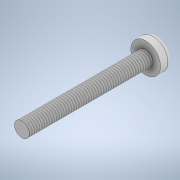
# Autodesk Inventor part: 16x2.5 Bolt
Saved by Autodesk Inventor 2022 (Build 260153000, 153)
## iProperties
Created: 2022-03-31
Part Number: 16x2.5 Bolt
Material: Generic
Document SubType Name: Modeling
Designer: Seppe
Density: 1 g/cm^3
Appearance: Default
Author: Seppe
Autodesk Inventor part; units mm, degrees
ref_plane "YZ Plane" through (0, 0, 0) normal (1, 0, 0) x (0, 1, 0)
ref_plane "XZ Plane" through (0, 0, 0) normal (0, 1, 0) x (-1, 0, 0)
ref_plane "XY Plane" through (0, 0, 0) normal (0, 0, 1) x (1, 0, 0)
sketch "Sketch1" plane through (0, 0, 0) normal (0, 0, 1) x (1, 0, 0)
  circle A0 centre (0, 0) radius 1.5
  circle A1 centre (0, 0) radius 3
  dimension "d0" = 3
  dimension "d1" = 6
  constraints: 2 centre point, 2 coincident
  measures "d0" diameter of A0
  measures "d1" diameter of A1
extrude "Extrusion1" add sketch "Sketch1" along normal blind 25 contours A0
sketch "Sketch2" plane through (0, 0, 0) normal (0, 0, -1) x (-1, 0, 0)
  point P0 (0, 0)
extrude "Extrusion2" add sketch "Sketch1" against normal blind 2.5 contours A0 | A1
thread "Thread1" size "M3x0.5" class "6g" standard "ISO Metric profile" full length
sketch "Sketch3" plane through (0, 0, -2.5) normal (0, 0, -1) x (-1, 0, 0)
  point P0 (0, 0)
sketch "Sketch4" plane through (0, 0, -2.5) normal (0, 0, -1) x (-1, 0, 0)
  line L0 (-0.5, -2) -> (0.5, -2)
  line L1 (0.5, -2) -> (0.5, 2)
  line L2 (0.5, 2) -> (-0.5, 2)
  line L3 (-0.5, 2) -> (-0.5, -2)
  circle A0 centre (0, 0) radius 1.5 projected
  line L4 (-0.5, -2) -> (0.5, 2) construction
  line L5 (0.5, -2) -> (-0.5, 2) construction
  line L6 (-2, -0.5) -> (2, -0.5)
  line L7 (2, -0.5) -> (2, 0.5)
  line L8 (2, 0.5) -> (-2, 0.5)
  line L9 (-2, 0.5) -> (-2, -0.5)
  circle A1 centre (0, 0) radius 3 projected
  line L10 (-2, -0.5) -> (2, 0.5) construction
  line L11 (2, -0.5) -> (-2, 0.5) construction
  point P0 (-0.5, 0.5)
  point P1 (-0.5, -0.5)
  point P2 (0.5, -0.5)
  point P3 (0.5, 0.5)
  dimension "d8" = 1
  dimension "d9" = 4
  dimension "d10" = 4
  dimension "d11" = 1
  constraints: 24 end point, 4 midpoint, 4 parallel, 2 horizontal, 2 perpendicular
  measures "d8" distance of L2.end L1.end
  measures "d9" distance of L1.end L0.end
  measures "d10" distance of L8.end L7.end
  measures "d11" distance of L7.end L6.end
extrude "Extrusion3" cut sketch "Sketch4" against normal blind 1 contours L3 A0 L1 L0 | L3 L6 L1 A0 | L6 A0 L8 L3 | L3 L8 L1 L6 | L6 L9 L8 A0 | L1 L8 A0 L6 | A0 L8 L7 L6 | L3 A0 L1 L8 | L3 L2 L1 A0
fillet "Fillet1" radius 1 1 edges at (-3, 0, -2.5)
body "Solid1"
